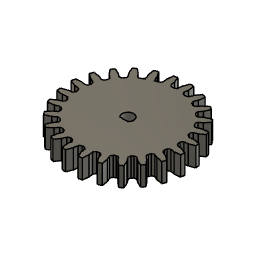
шестерня двигателя (Autodesk Fusion 360 design; units mm, degrees)
Autodesk Fusion 360 part; units mm, degrees
(part 1 of 2)
sketch "Sketch1" plane through (0, 0, 0) normal (0, 1, 0) x (1, 0, 0)
  circle A0 centre (0, 0) radius 12.5
  line L0 (0, 0) -> (0, 12.5)
  line L1 (0, 12.5) -> (0, 15.5)
  line L2 (0, 12.5) -> (-1.5967, 12.3976)
  line L3 (0, 0) -> (-1.5967, 12.3976)
  line L4 (-1.5967, 12.3976) -> (-1.9799, 15.373)
  line L5 (-1.9799, 15.373) -> (-3.666, 15.1559)
  line L6 (0, 12.5) -> (1.5967, 12.3976)
  line L7 (-3.666, 15.1559) -> (-3.268, 12.0653)
  line L8 (-4.751, 11.5619) -> (-5.8913, 14.3368)
  line L9 (-5.8913, 14.3368) -> (-7.4637, 13.6906)
  line L10 (-7.4637, 13.6906) -> (-6.2793, 10.8083)
  line L11 (-7.5816, 9.9383) -> (-9.4012, 12.3235)
  line L12 (-9.4012, 12.3235) -> (-10.7528, 11.2924)
  line L13 (-10.7528, 11.2924) -> (-8.8628, 8.8148)
  line L14 (-9.8955, 7.6374) -> (-12.2704, 9.4703)
  line L15 (-12.2704, 9.4703) -> (-13.3091, 8.1246)
  line L16 (-13.3091, 8.1246) -> (-10.8422, 6.2206)
  line L17 (-11.535, 4.816) -> (-14.3034, 5.9718)
  line L18 (-14.3034, 5.9718) -> (-14.9584, 4.4031)
  line L19 (-14.9584, 4.4031) -> (-12.0828, 3.2025)
  line L20 (-12.3884, 1.6664) -> (-15.3616, 2.0664)
  line L21 (-15.3616, 2.0664) -> (-15.5883, 0.3815)
  line L22 (-15.5883, 0.3815) -> (-12.5, -0.0339)
  line L23 (-12.3976, -1.5967) -> (-15.373, -1.9799)
  line L24 (-15.373, -1.9799) -> (-15.1559, -3.666)
  line L25 (-15.1559, -3.666) -> (-12.0653, -3.268)
  line L26 (-11.5619, -4.751) -> (-14.3368, -5.8913)
  line L27 (-14.3368, -5.8913) -> (-13.6906, -7.4637)
  line L28 (-13.6906, -7.4637) -> (-10.8083, -6.2793)
  line L29 (-9.9383, -7.5816) -> (-12.3235, -9.4012)
  line L30 (-12.3235, -9.4012) -> (-11.2924, -10.7528)
  line L31 (-11.2924, -10.7528) -> (-8.8148, -8.8628)
  line L32 (-7.6374, -9.8955) -> (-9.4703, -12.2704)
  line L33 (-9.4703, -12.2704) -> (-8.1246, -13.3091)
  line L34 (-8.1246, -13.3091) -> (-6.2206, -10.8422)
  line L35 (-4.816, -11.535) -> (-5.9718, -14.3034)
  line L36 (-5.9718, -14.3034) -> (-4.4031, -14.9584)
  line L37 (-4.4031, -14.9584) -> (-3.2025, -12.0828)
  line L38 (-1.6664, -12.3884) -> (-2.0664, -15.3616)
  line L39 (-2.0664, -15.3616) -> (-0.3815, -15.5883)
  line L40 (-0.3815, -15.5883) -> (0.0339, -12.5)
  line L41 (1.5967, -12.3976) -> (1.9799, -15.373)
  line L42 (1.9799, -15.373) -> (3.666, -15.1559)
  line L43 (3.666, -15.1559) -> (3.268, -12.0653)
  line L44 (4.751, -11.5619) -> (5.8913, -14.3368)
  line L45 (5.8913, -14.3368) -> (7.4637, -13.6906)
  line L46 (7.4637, -13.6906) -> (6.2793, -10.8083)
  line L47 (7.5816, -9.9383) -> (9.4012, -12.3235)
  line L48 (9.4012, -12.3235) -> (10.7528, -11.2924)
  line L49 (10.7528, -11.2924) -> (8.8628, -8.8148)
  line L50 (9.8955, -7.6374) -> (12.2704, -9.4703)
  line L51 (12.2704, -9.4703) -> (13.3091, -8.1246)
  line L52 (13.3091, -8.1246) -> (10.8422, -6.2206)
  line L53 (11.535, -4.816) -> (14.3034, -5.9718)
  line L54 (14.3034, -5.9718) -> (14.9584, -4.4031)
  line L55 (14.9584, -4.4031) -> (12.0828, -3.2025)
  line L56 (12.3884, -1.6664) -> (15.3616, -2.0664)
  line L57 (15.3616, -2.0664) -> (15.5883, -0.3815)
  line L58 (15.5883, -0.3815) -> (12.5, 0.0339)
  line L59 (12.3976, 1.5967) -> (15.373, 1.9799)
  line L60 (15.373, 1.9799) -> (15.1559, 3.666)
  line L61 (15.1559, 3.666) -> (12.0653, 3.268)
  line L62 (11.5619, 4.751) -> (14.3368, 5.8913)
  line L63 (14.3368, 5.8913) -> (13.6906, 7.4637)
  line L64 (13.6906, 7.4637) -> (10.8083, 6.2793)
  line L65 (9.9383, 7.5816) -> (12.3235, 9.4012)
  line L66 (12.3235, 9.4012) -> (11.2924, 10.7528)
  line L67 (11.2924, 10.7528) -> (8.8148, 8.8628)
  line L68 (7.6374, 9.8955) -> (9.4703, 12.2704)
  line L69 (9.4703, 12.2704) -> (8.1246, 13.3091)
  line L70 (8.1246, 13.3091) -> (6.2206, 10.8422)
  line L71 (4.816, 11.535) -> (5.9718, 14.3034)
  line L72 (5.9718, 14.3034) -> (4.4031, 14.9584)
  line L73 (4.4031, 14.9584) -> (3.2025, 12.0828)
  line L74 (1.6664, 12.3884) -> (2.0664, 15.3616)
  line L75 (2.0664, 15.3616) -> (0.3815, 15.5883)
  line L76 (0.3815, 15.5883) -> (-0.0339, 12.5)
  line L77 (-3.268, 12.0653) -> (-3.467, 13.6106)
  line L78 (-2.823, 15.2644) -> (-3.3189, 15.2006)
  line L79 (-2.823, 15.2644) -> (-2.3271, 15.3283)
  line L80 (-3.3189, 15.2006) -> (-3.467, 13.6106)
  line L81 (-2.3271, 15.3283) -> (-1.7883, 13.8853)
  line L82 (-6.215, 14.2037) -> (-5.3212, 12.9493)
  line L83 (-7.14, 13.8236) -> (-6.8715, 12.2495)
  line L84 (-9.6795, 12.1112) -> (-8.4914, 11.1309)
  line L85 (-10.4745, 11.5047) -> (-9.8078, 10.0536)
  line L86 (-12.4842, 9.1933) -> (-11.0829, 8.5539)
  line L87 (-13.0952, 8.4016) -> (-12.0756, 7.1726)
  line L88 (-14.4382, 5.6489) -> (-12.9192, 5.3939)
  line L89 (-14.8235, 4.7261) -> (-13.5206, 3.8028)
  line L90 (-15.4083, 1.7195) -> (-13.875, 1.8664)
  line L91 (-15.5416, 0.7284) -> (-14.0441, 0.1738)
  line L92 (-15.3283, -2.3271) -> (-13.8853, -1.7883)
  line L93 (-15.2006, -3.3189) -> (-13.6106, -3.467)
  line L94 (-14.2037, -6.215) -> (-12.9493, -5.3212)
  line L95 (-13.8236, -7.14) -> (-12.2495, -6.8715)
  line L96 (-12.1112, -9.6795) -> (-11.1309, -8.4914)
  line L97 (-11.5047, -10.4745) -> (-10.0536, -9.8078)
  line L98 (-9.1933, -12.4842) -> (-8.5539, -11.0829)
  line L99 (-8.4016, -13.0952) -> (-7.1726, -12.0756)
  line L100 (-5.6489, -14.4382) -> (-5.3939, -12.9192)
  line L101 (-4.7261, -14.8235) -> (-3.8028, -13.5206)
  line L102 (-1.7195, -15.4083) -> (-1.8664, -13.875)
  line L103 (-0.7284, -15.5416) -> (-0.1738, -14.0441)
  line L104 (2.3271, -15.3283) -> (1.7883, -13.8853)
  line L105 (3.3189, -15.2006) -> (3.467, -13.6106)
  line L106 (6.215, -14.2037) -> (5.3212, -12.9493)
  line L107 (7.14, -13.8236) -> (6.8715, -12.2495)
  line L108 (9.6795, -12.1112) -> (8.4914, -11.1309)
  line L109 (10.4745, -11.5047) -> (9.8078, -10.0536)
  line L110 (12.4842, -9.1933) -> (11.0829, -8.5539)
  line L111 (13.0952, -8.4016) -> (12.0756, -7.1726)
  line L112 (14.4382, -5.6489) -> (12.9192, -5.3939)
  line L113 (14.8235, -4.7261) -> (13.5206, -3.8028)
  line L114 (15.4083, -1.7195) -> (13.875, -1.8664)
  line L115 (15.5416, -0.7284) -> (14.0441, -0.1738)
  line L116 (15.3283, 2.3271) -> (13.8853, 1.7883)
  line L117 (15.2006, 3.3189) -> (13.6106, 3.467)
  line L118 (14.2037, 6.215) -> (12.9493, 5.3212)
  line L119 (13.8236, 7.14) -> (12.2495, 6.8715)
  line L120 (12.1112, 9.6795) -> (11.1309, 8.4914)
  line L121 (11.5047, 10.4745) -> (10.0536, 9.8078)
  line L122 (9.1933, 12.4842) -> (8.5539, 11.0829)
  line L123 (8.4016, 13.0952) -> (7.1726, 12.0756)
  line L124 (5.6489, 14.4382) -> (5.3939, 12.9192)
  line L125 (4.7261, 14.8235) -> (3.8028, 13.5206)
  line L126 (1.7195, 15.4083) -> (1.8664, 13.875)
  line L127 (0.7284, 15.5416) -> (0.1738, 14.0441)
  line L128 (-4.751, 11.5619) -> (-4.9411, 12.0244)
  line L129 (-4.751, 11.5619) -> (-4.2886, 11.7519)
  line L130 (-4.9411, 12.0244) -> (-4.2886, 11.7519)
  line L131 (-4.6148, 11.8882) -> (-4.6534, 11.7959)
  spline S0 degree 5 poles (-4.9411, 12.0244) (-4.931, 12.0121) (-4.9104, 11.9882) (-4.8789, 11.954) (-4.8353, 11.9119) (-4.778, 11.8656) (-4.7177, 11.8261) (-4.6541, 11.7939) (-4.5872, 11.7695) (-4.517, 11.7524) (-4.4438, 11.7421) (-4.383, 11.7389) (-4.3362, 11.7391) (-4.3045, 11.7404) (-4.2886, 11.7413) knots 0 0 0 0 0 0 0.1 0.2 0.3 0.4 0.5 0.6 0.7 0.8 0.9 1 1 1 1 1 1
  line L132 (-6.2793, 10.8083) -> (-6.4694, 11.2708)
  line L133 (-6.2793, 10.8083) -> (-6.7117, 10.5572)
  line L134 (-6.4694, 11.2708) -> (-6.7117, 10.5572)
  line L135 (-6.5905, 10.914) -> (-6.4958, 10.8818)
  spline S1 degree 5 poles (-6.4694, 11.2708) (-6.467, 11.2543) (-6.4628, 11.2214) (-6.4584, 11.1727) (-6.4566, 11.1087) (-6.4612, 11.0305) (-6.4735, 10.9543) (-6.494, 10.8803) (-6.523, 10.8086) (-6.5603, 10.739) (-6.6051, 10.6714) (-6.6465, 10.6188) (-6.6805, 10.5801) (-6.7045, 10.5547) (-6.7168, 10.542) knots 0 0 0 0 0 0 0.1 0.2 0.3 0.4 0.5 0.6 0.7 0.8 0.9 1 1 1 1 1 1
  spline S2 degree 5 poles (-7.8849, 10.3358) (-7.8719, 10.3266) (-7.8459, 10.3088) (-7.8066, 10.2839) (-7.7535, 10.2546) (-7.6862, 10.2246) (-7.6177, 10.2021) (-7.548, 10.1875) (-7.477, 10.1812) (-7.4048, 10.1828) (-7.3314, 10.1918) (-7.2719, 10.2045) (-7.2268, 10.2168) (-7.1965, 10.2262) (-7.1813, 10.2313) knots 0 0 0 0 0 0 0.1 0.2 0.3 0.4 0.5 0.6 0.7 0.8 0.9 1 1 1 1 1 1
  spline S3 degree 5 poles (-9.166, 9.2124) (-9.1594, 9.197) (-9.1469, 9.1664) (-9.1301, 9.1204) (-9.1117, 9.0591) (-9.096, 8.9823) (-9.0881, 8.9056) (-9.0888, 8.8288) (-9.0982, 8.752) (-9.1162, 8.6752) (-9.142, 8.5983) (-9.1684, 8.5367) (-9.1913, 8.4906) (-9.2078, 8.4598) (-9.2164, 8.4444) knots 0 0 0 0 0 0 0.1 0.2 0.3 0.4 0.5 0.6 0.7 0.8 0.9 1 1 1 1 1 1
  spline S4 degree 5 poles (-10.2913, 7.9429) (-10.2764, 7.9373) (-10.2466, 7.9268) (-10.2022, 7.913) (-10.1434, 7.8984) (-10.0706, 7.8869) (-9.9987, 7.8828) (-9.9276, 7.8868) (-9.8573, 7.8991) (-9.788, 7.9194) (-9.7194, 7.9471) (-9.6652, 7.9747) (-9.6248, 7.9982) (-9.598, 8.0152) (-9.5847, 8.024) knots 0 0 0 0 0 0 0.1 0.2 0.3 0.4 0.5 0.6 0.7 0.8 0.9 1 1 1 1 1 1
  spline S5 degree 5 poles (-11.238, 6.5261) (-11.2277, 6.513) (-11.2076, 6.4867) (-11.1795, 6.4466) (-11.1459, 6.3921) (-11.1109, 6.3221) (-11.0834, 6.25) (-11.0641, 6.1756) (-11.0534, 6.099) (-11.0509, 6.0201) (-11.0559, 5.9392) (-11.0655, 5.8729) (-11.0756, 5.8224) (-11.0836, 5.7884) (-11.0879, 5.7713) knots 0 0 0 0 0 0 0.1 0.2 0.3 0.4 0.5 0.6 0.7 0.8 0.9 1 1 1 1 1 1
  spline S6 degree 5 poles (-11.9964, 5.0086) (-11.9806, 5.0071) (-11.9491, 5.0047) (-11.9026, 5.0029) (-11.842, 5.0039) (-11.7688, 5.0117) (-11.6982, 5.0264) (-11.6305, 5.0486) (-11.5659, 5.0786) (-11.5042, 5.1162) (-11.4451, 5.1607) (-11.3998, 5.2014) (-11.3669, 5.2346) (-11.3455, 5.2579) (-11.3348, 5.2699) knots 0 0 0 0 0 0 0.1 0.2 0.3 0.4 0.5 0.6 0.7 0.8 0.9 1 1 1 1 1 1
  spline S7 degree 5 poles (-12.5442, 3.3951) (-12.5308, 3.3852) (-12.5046, 3.3649) (-12.4671, 3.3335) (-12.4205, 3.2895) (-12.3685, 3.2309) (-12.3233, 3.1684) (-12.2855, 3.1016) (-12.2553, 3.0303) (-12.2325, 2.9548) (-12.2164, 2.8753) (-12.2085, 2.8088) (-12.2051, 2.7574) (-12.2041, 2.7225) (-12.2038, 2.7049) knots 0 0 0 0 0 0 0.1 0.2 0.3 0.4 0.5 0.6 0.7 0.8 0.9 1 1 1 1 1 1
  spline S8 degree 5 poles (-12.884, 1.7331) (-12.8683, 1.7357) (-12.8373, 1.7415) (-12.7919, 1.7518) (-12.7337, 1.7685) (-12.6649, 1.7949) (-12.6005, 1.8274) (-12.5409, 1.8664) (-12.4862, 1.9121) (-12.4363, 1.9644) (-12.3908, 2.0226) (-12.3576, 2.0737) (-12.3344, 2.1143) (-12.3197, 2.1423) (-12.3126, 2.1566) knots 0 0 0 0 0 0 0.1 0.2 0.3 0.4 0.5 0.6 0.7 0.8 0.9 1 1 1 1 1 1
  spline S9 degree 5 poles (-12.9955, 0.0328) (-12.98, 0.0266) (-12.9494, 0.0138) (-12.905, -0.0068) (-12.8487, -0.0372) (-12.7833, -0.0804) (-12.7235, -0.1291) (-12.6697, -0.1838) (-12.622, -0.2448) (-12.5804, -0.3119) (-12.5443, -0.3845) (-12.5194, -0.4467) (-12.5029, -0.4955) (-12.4929, -0.5289) (-12.4881, -0.5459) knots 0 0 0 0 0 0 0.1 0.2 0.3 0.4 0.5 0.6 0.7 0.8 0.9 1 1 1 1 1 1
  spline S10 degree 5 poles (-12.8935, -1.6606) (-12.879, -1.654) (-12.8506, -1.6403) (-12.8094, -1.6187) (-12.7575, -1.5875) (-12.6979, -1.5441) (-12.6441, -1.4961) (-12.5966, -1.443) (-12.5557, -1.3847) (-12.521, -1.3213) (-12.4921, -1.2533) (-12.4733, -1.1954) (-12.4614, -1.1502) (-12.4544, -1.1192) (-12.4512, -1.1036) knots 0 0 0 0 0 0 0.1 0.2 0.3 0.4 0.5 0.6 0.7 0.8 0.9 1 1 1 1 1 1
  spline S11 degree 5 poles (-12.5612, -3.3318) (-12.5446, -3.3338) (-12.5118, -3.3382) (-12.4635, -3.3467) (-12.4012, -3.3614) (-12.3269, -3.3862) (-12.2565, -3.4177) (-12.1904, -3.4567) (-12.1286, -3.5033) (-12.071, -3.5573) (-12.0173, -3.6181) (-11.9772, -3.6717) (-11.9487, -3.7146) (-11.9303, -3.7443) (-11.9213, -3.7594) knots 0 0 0 0 0 0 0.1 0.2 0.3 0.4 0.5 0.6 0.7 0.8 0.9 1 1 1 1 1 1
  spline S12 degree 5 poles (-12.0244, -4.9411) (-12.0121, -4.931) (-11.9882, -4.9104) (-11.954, -4.8789) (-11.9119, -4.8353) (-11.8656, -4.778) (-11.8261, -4.7177) (-11.7939, -4.6541) (-11.7695, -4.5872) (-11.7524, -4.517) (-11.7421, -4.4438) (-11.7389, -4.383) (-11.7391, -4.3362) (-11.7404, -4.3045) (-11.7413, -4.2886) knots 0 0 0 0 0 0 0.1 0.2 0.3 0.4 0.5 0.6 0.7 0.8 0.9 1 1 1 1 1 1
  spline S13 degree 5 poles (-11.2708, -6.4694) (-11.2543, -6.467) (-11.2214, -6.4628) (-11.1727, -6.4584) (-11.1087, -6.4566) (-11.0305, -6.4612) (-10.9543, -6.4735) (-10.8803, -6.494) (-10.8086, -6.523) (-10.739, -6.5603) (-10.6714, -6.6051) (-10.6188, -6.6465) (-10.5801, -6.6805) (-10.5547, -6.7045) (-10.542, -6.7168) knots 0 0 0 0 0 0 0.1 0.2 0.3 0.4 0.5 0.6 0.7 0.8 0.9 1 1 1 1 1 1
  spline S14 degree 5 poles (-10.3358, -7.8849) (-10.3266, -7.8719) (-10.3088, -7.8459) (-10.2839, -7.8066) (-10.2546, -7.7535) (-10.2246, -7.6862) (-10.2021, -7.6177) (-10.1875, -7.548) (-10.1812, -7.477) (-10.1828, -7.4048) (-10.1918, -7.3314) (-10.2045, -7.2719) (-10.2168, -7.2268) (-10.2262, -7.1965) (-10.2313, -7.1813) knots 0 0 0 0 0 0 0.1 0.2 0.3 0.4 0.5 0.6 0.7 0.8 0.9 1 1 1 1 1 1
  spline S15 degree 5 poles (-9.2124, -9.166) (-9.197, -9.1594) (-9.1664, -9.1469) (-9.1204, -9.1301) (-9.0591, -9.1117) (-8.9823, -9.096) (-8.9056, -9.0881) (-8.8288, -9.0888) (-8.752, -9.0982) (-8.6752, -9.1162) (-8.5983, -9.142) (-8.5367, -9.1684) (-8.4906, -9.1913) (-8.4598, -9.2078) (-8.4444, -9.2164) knots 0 0 0 0 0 0 0.1 0.2 0.3 0.4 0.5 0.6 0.7 0.8 0.9 1 1 1 1 1 1
  spline S16 degree 5 poles (-7.9429, -10.2913) (-7.9373, -10.2764) (-7.9268, -10.2466) (-7.913, -10.2022) (-7.8984, -10.1434) (-7.8869, -10.0706) (-7.8828, -9.9987) (-7.8868, -9.9276) (-7.8991, -9.8573) (-7.9194, -9.788) (-7.9471, -9.7194) (-7.9747, -9.6652) (-7.9982, -9.6248) (-8.0152, -9.598) (-8.024, -9.5847) knots 0 0 0 0 0 0 0.1 0.2 0.3 0.4 0.5 0.6 0.7 0.8 0.9 1 1 1 1 1 1
  spline S17 degree 5 poles (-6.5261, -11.238) (-6.513, -11.2277) (-6.4867, -11.2076) (-6.4466, -11.1795) (-6.3921, -11.1459) (-6.3221, -11.1109) (-6.25, -11.0834) (-6.1756, -11.0641) (-6.099, -11.0534) (-6.0201, -11.0509) (-5.9392, -11.0559) (-5.8729, -11.0655) (-5.8224, -11.0756) (-5.7884, -11.0836) (-5.7713, -11.0879) knots 0 0 0 0 0 0 0.1 0.2 0.3 0.4 0.5 0.6 0.7 0.8 0.9 1 1 1 1 1 1
  spline S18 degree 5 poles (-5.0086, -11.9964) (-5.0071, -11.9806) (-5.0047, -11.9491) (-5.0029, -11.9026) (-5.0039, -11.842) (-5.0117, -11.7688) (-5.0264, -11.6982) (-5.0486, -11.6305) (-5.0786, -11.5659) (-5.1162, -11.5042) (-5.1607, -11.4451) (-5.2014, -11.3998) (-5.2346, -11.3669) (-5.2579, -11.3455) (-5.2699, -11.3348) knots 0 0 0 0 0 0 0.1 0.2 0.3 0.4 0.5 0.6 0.7 0.8 0.9 1 1 1 1 1 1
  spline S19 degree 5 poles (-3.3951, -12.5442) (-3.3852, -12.5308) (-3.3649, -12.5046) (-3.3335, -12.4671) (-3.2895, -12.4205) (-3.2309, -12.3685) (-3.1684, -12.3233) (-3.1016, -12.2855) (-3.0303, -12.2553) (-2.9548, -12.2325) (-2.8753, -12.2164) (-2.8088, -12.2085) (-2.7574, -12.2051) (-2.7225, -12.2041) (-2.7049, -12.2038) knots 0 0 0 0 0 0 0.1 0.2 0.3 0.4 0.5 0.6 0.7 0.8 0.9 1 1 1 1 1 1
  spline S20 degree 5 poles (-1.7331, -12.884) (-1.7357, -12.8683) (-1.7415, -12.8373) (-1.7518, -12.7919) (-1.7685, -12.7337) (-1.7949, -12.6649) (-1.8274, -12.6005) (-1.8664, -12.5409) (-1.9121, -12.4862) (-1.9644, -12.4363) (-2.0226, -12.3908) (-2.0737, -12.3576) (-2.1143, -12.3344) (-2.1423, -12.3197) (-2.1566, -12.3126) knots 0 0 0 0 0 0 0.1 0.2 0.3 0.4 0.5 0.6 0.7 0.8 0.9 1 1 1 1 1 1
  spline S21 degree 5 poles (-0.0328, -12.9955) (-0.0266, -12.98) (-0.0138, -12.9494) (0.0068, -12.905) (0.0372, -12.8487) (0.0804, -12.7833) (0.1291, -12.7235) (0.1838, -12.6697) (0.2448, -12.622) (0.3119, -12.5804) (0.3845, -12.5443) (0.4467, -12.5194) (0.4955, -12.5029) (0.5289, -12.4929) (0.5459, -12.4881) knots 0 0 0 0 0 0 0.1 0.2 0.3 0.4 0.5 0.6 0.7 0.8 0.9 1 1 1 1 1 1
  spline S22 degree 5 poles (1.6606, -12.8935) (1.654, -12.879) (1.6403, -12.8506) (1.6187, -12.8094) (1.5875, -12.7575) (1.5441, -12.6979) (1.4961, -12.6441) (1.443, -12.5966) (1.3847, -12.5557) (1.3213, -12.521) (1.2533, -12.4921) (1.1954, -12.4733) (1.1502, -12.4614) (1.1192, -12.4544) (1.1036, -12.4512) knots 0 0 0 0 0 0 0.1 0.2 0.3 0.4 0.5 0.6 0.7 0.8 0.9 1 1 1 1 1 1
  spline S23 degree 5 poles (3.3318, -12.5612) (3.3338, -12.5446) (3.3382, -12.5118) (3.3467, -12.4635) (3.3614, -12.4012) (3.3862, -12.3269) (3.4177, -12.2565) (3.4567, -12.1904) (3.5033, -12.1286) (3.5573, -12.071) (3.6181, -12.0173) (3.6717, -11.9772) (3.7146, -11.9487) (3.7443, -11.9303) (3.7594, -11.9213) knots 0 0 0 0 0 0 0.1 0.2 0.3 0.4 0.5 0.6 0.7 0.8 0.9 1 1 1 1 1 1
  spline S24 degree 5 poles (4.9411, -12.0244) (4.931, -12.0121) (4.9104, -11.9882) (4.8789, -11.954) (4.8353, -11.9119) (4.778, -11.8656) (4.7177, -11.8261) (4.6541, -11.7939) (4.5872, -11.7695) (4.517, -11.7524) (4.4438, -11.7421) (4.383, -11.7389) (4.3362, -11.7391) (4.3045, -11.7404) (4.2886, -11.7413) knots 0 0 0 0 0 0 0.1 0.2 0.3 0.4 0.5 0.6 0.7 0.8 0.9 1 1 1 1 1 1
  spline S25 degree 5 poles (6.4694, -11.2708) (6.467, -11.2543) (6.4628, -11.2214) (6.4584, -11.1727) (6.4566, -11.1087) (6.4612, -11.0305) (6.4735, -10.9543) (6.494, -10.8803) (6.523, -10.8086) (6.5603, -10.739) (6.6051, -10.6714) (6.6465, -10.6188) (6.6805, -10.5801) (6.7045, -10.5547) (6.7168, -10.542) knots 0 0 0 0 0 0 0.1 0.2 0.3 0.4 0.5 0.6 0.7 0.8 0.9 1 1 1 1 1 1
  spline S26 degree 5 poles (7.8849, -10.3358) (7.8719, -10.3266) (7.8459, -10.3088) (7.8066, -10.2839) (7.7535, -10.2546) (7.6862, -10.2246) (7.6177, -10.2021) (7.548, -10.1875) (7.477, -10.1812) (7.4048, -10.1828) (7.3314, -10.1918) (7.2719, -10.2045) (7.2268, -10.2168) (7.1965, -10.2262) (7.1813, -10.2313) knots 0 0 0 0 0 0 0.1 0.2 0.3 0.4 0.5 0.6 0.7 0.8 0.9 1 1 1 1 1 1
  spline S27 degree 5 poles (9.166, -9.2124) (9.1594, -9.197) (9.1469, -9.1664) (9.1301, -9.1204) (9.1117, -9.0591) (9.096, -8.9823) (9.0881, -8.9056) (9.0888, -8.8288) (9.0982, -8.752) (9.1162, -8.6752) (9.142, -8.5983) (9.1684, -8.5367) (9.1913, -8.4906) (9.2078, -8.4598) (9.2164, -8.4444) knots 0 0 0 0 0 0 0.1 0.2 0.3 0.4 0.5 0.6 0.7 0.8 0.9 1 1 1 1 1 1
  spline S28 degree 5 poles (10.2913, -7.9429) (10.2764, -7.9373) (10.2466, -7.9268) (10.2022, -7.913) (10.1434, -7.8984) (10.0706, -7.8869) (9.9987, -7.8828) (9.9276, -7.8868) (9.8573, -7.8991) (9.788, -7.9194) (9.7194, -7.9471) (9.6652, -7.9747) (9.6248, -7.9982) (9.598, -8.0152) (9.5847, -8.024) knots 0 0 0 0 0 0 0.1 0.2 0.3 0.4 0.5 0.6 0.7 0.8 0.9 1 1 1 1 1 1
  spline S29 degree 5 poles (11.238, -6.5261) (11.2277, -6.513) (11.2076, -6.4867) (11.1795, -6.4466) (11.1459, -6.3921) (11.1109, -6.3221) (11.0834, -6.25) (11.0641, -6.1756) (11.0534, -6.099) (11.0509, -6.0201) (11.0559, -5.9392) (11.0655, -5.8729) (11.0756, -5.8224) (11.0836, -5.7884) (11.0879, -5.7713) knots 0 0 0 0 0 0 0.1 0.2 0.3 0.4 0.5 0.6 0.7 0.8 0.9 1 1 1 1 1 1
  spline S30 degree 5 poles (11.9964, -5.0086) (11.9806, -5.0071) (11.9491, -5.0047) (11.9026, -5.0029) (11.842, -5.0039) (11.7688, -5.0117) (11.6982, -5.0264) (11.6305, -5.0486) (11.5659, -5.0786) (11.5042, -5.1162) (11.4451, -5.1607) (11.3998, -5.2014) (11.3669, -5.2346) (11.3455, -5.2579) (11.3348, -5.2699) knots 0 0 0 0 0 0 0.1 0.2 0.3 0.4 0.5 0.6 0.7 0.8 0.9 1 1 1 1 1 1
  spline S31 degree 5 poles (12.5442, -3.3951) (12.5308, -3.3852) (12.5046, -3.3649) (12.4671, -3.3335) (12.4205, -3.2895) (12.3685, -3.2309) (12.3233, -3.1684) (12.2855, -3.1016) (12.2553, -3.0303) (12.2325, -2.9548) (12.2164, -2.8753) (12.2085, -2.8088) (12.2051, -2.7574) (12.2041, -2.7225) (12.2038, -2.7049) knots 0 0 0 0 0 0 0.1 0.2 0.3 0.4 0.5 0.6 0.7 0.8 0.9 1 1 1 1 1 1
  spline S32 degree 5 poles (12.884, -1.7331) (12.8683, -1.7357) (12.8373, -1.7415) (12.7919, -1.7518) (12.7337, -1.7685) (12.6649, -1.7949) (12.6005, -1.8274) (12.5409, -1.8664) (12.4862, -1.9121) (12.4363, -1.9644) (12.3908, -2.0226) (12.3576, -2.0737) (12.3344, -2.1143) (12.3197, -2.1423) (12.3126, -2.1566) knots 0 0 0 0 0 0 0.1 0.2 0.3 0.4 0.5 0.6 0.7 0.8 0.9 1 1 1 1 1 1
  spline S33 degree 5 poles (12.9955, -0.0328) (12.98, -0.0266) (12.9494, -0.0138) (12.905, 0.0068) (12.8487, 0.0372) (12.7833, 0.0804) (12.7235, 0.1291) (12.6697, 0.1838) (12.622, 0.2448) (12.5804, 0.3119) (12.5443, 0.3845) (12.5194, 0.4467) (12.5029, 0.4955) (12.4929, 0.5289) (12.4881, 0.5459) knots 0 0 0 0 0 0 0.1 0.2 0.3 0.4 0.5 0.6 0.7 0.8 0.9 1 1 1 1 1 1
  spline S34 degree 5 poles (12.8935, 1.6606) (12.879, 1.654) (12.8506, 1.6403) (12.8094, 1.6187) (12.7575, 1.5875) (12.6979, 1.5441) (12.6441, 1.4961) (12.5966, 1.443) (12.5557, 1.3847) (12.521, 1.3213) (12.4921, 1.2533) (12.4733, 1.1954) (12.4614, 1.1502) (12.4544, 1.1192) (12.4512, 1.1036) knots 0 0 0 0 0 0 0.1 0.2 0.3 0.4 0.5 0.6 0.7 0.8 0.9 1 1 1 1 1 1
  spline S35 degree 5 poles (12.5612, 3.3318) (12.5446, 3.3338) (12.5118, 3.3382) (12.4635, 3.3467) (12.4012, 3.3614) (12.3269, 3.3862) (12.2565, 3.4177) (12.1904, 3.4567) (12.1286, 3.5033) (12.071, 3.5573) (12.0173, 3.6181) (11.9772, 3.6717) (11.9487, 3.7146) (11.9303, 3.7443) (11.9213, 3.7594) knots 0 0 0 0 0 0 0.1 0.2 0.3 0.4 0.5 0.6 0.7 0.8 0.9 1 1 1 1 1 1
  spline S36 degree 5 poles (12.0244, 4.9411) (12.0121, 4.931) (11.9882, 4.9104) (11.954, 4.8789) (11.9119, 4.8353) (11.8656, 4.778) (11.8261, 4.7177) (11.7939, 4.6541) (11.7695, 4.5872) (11.7524, 4.517) (11.7421, 4.4438) (11.7389, 4.383) (11.7391, 4.3362) (11.7404, 4.3045) (11.7413, 4.2886) knots 0 0 0 0 0 0 0.1 0.2 0.3 0.4 0.5 0.6 0.7 0.8 0.9 1 1 1 1 1 1
  spline S37 degree 5 poles (11.2708, 6.4694) (11.2543, 6.467) (11.2214, 6.4628) (11.1727, 6.4584) (11.1087, 6.4566) (11.0305, 6.4612) (10.9543, 6.4735) (10.8803, 6.494) (10.8086, 6.523) (10.739, 6.5603) (10.6714, 6.6051) (10.6188, 6.6465) (10.5801, 6.6805) (10.5547, 6.7045) (10.542, 6.7168) knots 0 0 0 0 0 0 0.1 0.2 0.3 0.4 0.5 0.6 0.7 0.8 0.9 1 1 1 1 1 1
  spline S38 degree 5 poles (10.3358, 7.8849) (10.3266, 7.8719) (10.3088, 7.8459) (10.2839, 7.8066) (10.2546, 7.7535) (10.2246, 7.6862) (10.2021, 7.6177) (10.1875, 7.548) (10.1812, 7.477) (10.1828, 7.4048) (10.1918, 7.3314) (10.2045, 7.2719) (10.2168, 7.2268) (10.2262, 7.1965) (10.2313, 7.1813) knots 0 0 0 0 0 0 0.1 0.2 0.3 0.4 0.5 0.6 0.7 0.8 0.9 1 1 1 1 1 1
  spline S39 degree 5 poles (9.2124, 9.166) (9.197, 9.1594) (9.1664, 9.1469) (9.1204, 9.1301) (9.0591, 9.1117) (8.9823, 9.096) (8.9056, 9.0881) (8.8288, 9.0888) (8.752, 9.0982) (8.6752, 9.1162) (8.5983, 9.142) (8.5367, 9.1684) (8.4906, 9.1913) (8.4598, 9.2078) (8.4444, 9.2164) knots 0 0 0 0 0 0 0.1 0.2 0.3 0.4 0.5 0.6 0.7 0.8 0.9 1 1 1 1 1 1
  spline S40 degree 5 poles (7.9429, 10.2913) (7.9373, 10.2764) (7.9268, 10.2466) (7.913, 10.2022) (7.8984, 10.1434) (7.8869, 10.0706) (7.8828, 9.9987) (7.8868, 9.9276) (7.8991, 9.8573) (7.9194, 9.788) (7.9471, 9.7194) (7.9747, 9.6652) (7.9982, 9.6248) (8.0152, 9.598) (8.024, 9.5847) knots 0 0 0 0 0 0 0.1 0.2 0.3 0.4 0.5 0.6 0.7 0.8 0.9 1 1 1 1 1 1
  spline S41 degree 5 poles (6.5261, 11.238) (6.513, 11.2277) (6.4867, 11.2076) (6.4466, 11.1795) (6.3921, 11.1459) (6.3221, 11.1109) (6.25, 11.0834) (6.1756, 11.0641) (6.099, 11.0534) (6.0201, 11.0509) (5.9392, 11.0559) (5.8729, 11.0655) (5.8224, 11.0756) (5.7884, 11.0836) (5.7713, 11.0879) knots 0 0 0 0 0 0 0.1 0.2 0.3 0.4 0.5 0.6 0.7 0.8 0.9 1 1 1 1 1 1
  spline S42 degree 5 poles (5.0086, 11.9964) (5.0071, 11.9806) (5.0047, 11.9491) (5.0029, 11.9026) (5.0039, 11.842) (5.0117, 11.7688) (5.0264, 11.6982) (5.0486, 11.6305) (5.0786, 11.5659) (5.1162, 11.5042) (5.1607, 11.4451) (5.2014, 11.3998) (5.2346, 11.3669) (5.2579, 11.3455) (5.2699, 11.3348) knots 0 0 0 0 0 0 0.1 0.2 0.3 0.4 0.5 0.6 0.7 0.8 0.9 1 1 1 1 1 1
  spline S43 degree 5 poles (3.3951, 12.5442) (3.3852, 12.5308) (3.3649, 12.5046) (3.3335, 12.4671) (3.2895, 12.4205) (3.2309, 12.3685) (3.1684, 12.3233) (3.1016, 12.2855) (3.0303, 12.2553) (2.9548, 12.2325) (2.8753, 12.2164) (2.8088, 12.2085) (2.7574, 12.2051) (2.7225, 12.2041) (2.7049, 12.2038) knots 0 0 0 0 0 0 0.1 0.2 0.3 0.4 0.5 0.6 0.7 0.8 0.9 1 1 1 1 1 1
  spline S44 degree 5 poles (1.7331, 12.884) (1.7357, 12.8683) (1.7415, 12.8373) (1.7518, 12.7919) (1.7685, 12.7337) (1.7949, 12.6649) (1.8274, 12.6005) (1.8664, 12.5409) (1.9121, 12.4862) (1.9644, 12.4363) (2.0226, 12.3908) (2.0737, 12.3576) (2.1143, 12.3344) (2.1423, 12.3197) (2.1566, 12.3126) knots 0 0 0 0 0 0 0.1 0.2 0.3 0.4 0.5 0.6 0.7 0.8 0.9 1 1 1 1 1 1
  spline S45 degree 5 poles (0.0328, 12.9955) (0.0266, 12.98) (0.0138, 12.9494) (-0.0068, 12.905) (-0.0372, 12.8487) (-0.0804, 12.7833) (-0.1291, 12.7235) (-0.1838, 12.6697) (-0.2448, 12.622) (-0.3119, 12.5804) (-0.3845, 12.5443) (-0.4467, 12.5194) (-0.4955, 12.5029) (-0.5289, 12.4929) (-0.5459, 12.4881) knots 0 0 0 0 0 0 0.1 0.2 0.3 0.4 0.5 0.6 0.7 0.8 0.9 1 1 1 1 1 1
  spline S46 degree 5 poles (-1.6606, 12.8935) (-1.654, 12.879) (-1.6403, 12.8506) (-1.6187, 12.8094) (-1.5875, 12.7575) (-1.5441, 12.6979) (-1.4961, 12.6441) (-1.443, 12.5966) (-1.3847, 12.5557) (-1.3213, 12.521) (-1.2533, 12.4921) (-1.1954, 12.4733) (-1.1502, 12.4614) (-1.1192, 12.4544) (-1.1036, 12.4512) knots 0 0 0 0 0 0 0.1 0.2 0.3 0.4 0.5 0.6 0.7 0.8 0.9 1 1 1 1 1 1
  spline S47 degree 5 poles (-3.3318, 12.5612) (-3.3338, 12.5446) (-3.3382, 12.5118) (-3.3467, 12.4635) (-3.3614, 12.4012) (-3.3862, 12.3269) (-3.4177, 12.2565) (-3.4567, 12.1904) (-3.5033, 12.1286) (-3.5573, 12.071) (-3.6181, 12.0173) (-3.6717, 11.9772) (-3.7146, 11.9487) (-3.7443, 11.9303) (-3.7594, 11.9213) knots 0 0 0 0 0 0 0.1 0.2 0.3 0.4 0.5 0.6 0.7 0.8 0.9 1 1 1 1 1 1
  point P0 (-7.5478, 10.1896)
  point P1 (-9.0909, 8.8298)
  point P2 (-9.9279, 7.8889)
  point P3 (-11.0665, 6.176)
  point P4 (-11.6314, 5.0505)
  point P5 (-12.2879, 3.1014)
  point P6 (-12.5422, 1.868)
  point P7 (-12.6719, -0.1846)
  point P8 (-12.5983, -1.4418)
  point P9 (-12.1923, -3.4581)
  point P10 (-11.7959, -4.6534)
  point P11 (-10.8818, -6.4958)
  point P12 (-10.1896, -7.5478)
  point P13 (-8.8298, -9.0909)
  point P14 (-7.8889, -9.9279)
  point P15 (-6.176, -11.0665)
  point P16 (-5.0505, -11.6314)
  point P17 (-3.1014, -12.2879)
  point P18 (-1.868, -12.5422)
  point P19 (0.1846, -12.6719)
  point P20 (1.4418, -12.5983)
  point P21 (3.4581, -12.1923)
  point P22 (4.6534, -11.7959)
  point P23 (6.4958, -10.8818)
  point P24 (7.5478, -10.1896)
  point P25 (9.0909, -8.8298)
  point P26 (9.9279, -7.8889)
  point P27 (11.0665, -6.176)
  point P28 (11.6314, -5.0505)
  point P29 (12.2879, -3.1014)
  point P30 (12.5422, -1.868)
  point P31 (12.6719, 0.1846)
  point P32 (12.5983, 1.4418)
  point P33 (12.1923, 3.4581)
  point P34 (11.7959, 4.6534)
  point P35 (10.8818, 6.4958)
  point P36 (10.1896, 7.5478)
  point P37 (8.8298, 9.0909)
  point P38 (7.8889, 9.9279)
  point P39 (6.176, 11.0665)
  point P40 (5.0505, 11.6314)
  point P41 (3.1014, 12.2879)
  point P42 (1.868, 12.5422)
  point P43 (-0.1846, 12.6719)
  point P44 (-1.4418, 12.5983)
  point P45 (-3.4581, 12.1923)
  dimension "d1" = 25
  dimension "d2" = 3
  dimension "d3" = 1.6
  dimension "d4" = 3
  dimension "d5" = 1.7
  dimension "d6" = 1.6
  dimension "d8" = 360
  dimension "d9" = 0.5
  dimension "d10" = 0.5
  dimension "d12" = 360
  dimension "d13" = 0.5
  dimension "d14" = 0.5
  dimension "d15" = 0.1
  dimension "d16" = 0.5
  dimension "d17" = 0.5
  dimension "d18" = 0.1
  dimension "d20" = 360
  constraint coincident A0.centre L0.start
  constraint coincident A0 L0.end
  constraint vertical L0
  constraint parallel L0 L1
  constraint coincident A0 L2.end
  constraint parallel L3 L4
  constraint perpendicular L4 L5
  constraint coincident A0 L6.end
  constraint coincident A0 L7.end
  constraint perpendicular L5 L7
  constraint midpoint L7 L77.end
  constraint midpoint L5 L78.start
  constraint parallel L5 L78
  constraint parallel L5 L79
  constraint midpoint L4 L81.end
  constraint parallel L8 L128
  constraint perpendicular L8 L129
  constraint midpoint L130 L131.start
  constraint perpendicular L130 L131
  constraint coincident A0 S0.end
  constraint parallel L10 L132
  constraint tangent A0 L133
  constraint midpoint L134 L135.start
  constraint perpendicular L134 L135
  constraint coincident A0 S1.end
  measures "d1" diameter of A0
  measures "d2" distance of L0.end L1.end
  measures "d3" distance of L0.end L2.end
  measures "d4" distance of L2.end L4.end
  measures "d5" distance of L4.end L5.end
  measures "d6" distance of L0.end L6.end
  measures "d9" distance of L78.start L78.end
  measures "d10" distance of L78.start L79.end
  measures "d13" distance of L8.start L128.end
  measures "d14" distance of L8.start L129.end
  measures "d15" distance of L131.start L131.end
  measures "d16" distance of L10.end L132.end
  measures "d17" distance of L10.end L133.end
  measures "d18" distance of L135.start L135.end
extrude "Extrude1" add sketch "Sketch1" along normal blind 4 contours A0 L0 L3 L6 | A0 L56 L57 L58 L114 L115 | A0 L58 S33 | A0 L56 S32 | A0 L59 S34 | A0 L55 S31 | A0 L59 L60 L61 L116 L117 | A0 L53 L54 L55 L112 L113 | A0 L61 S35 | A0 L53 S30 | A0 L62 S36 | A0 L52 S29 | A0 L62 L63 L64 L118 L119 | A0 L50 L51 L52 L110 L111 | A0 L64 S37 | A0 L50 S28 | A0 L65 S38 | A0 L49 S27 | A0 L65 L66 L67 L120 L121 | A0 L47 L48 L49 L108 L109 | A0 L67 S39 | A0 L47 S26 | A0 L68 S40 | A0 L46 S25 | A0 L68 L69 L70 L122 L123 | A0 L44 L45 L46 L106 L107 | A0 L70 S41 | A0 L44 S24 | A0 L71 S42 | A0 L43 S23 | A0 L71 L72 L73 L124 L125 | A0 L41 L42 L43 L104 L105 | A0 L73 S43 | A0 L41 S22 | A0 L74 S44 | A0 L40 S21 | A0 L1 L74 L75 L76 L126 L127 | A0 L38 L39 L40 L102 L103 | A0 L6 | A0 L38 S20 | A0 L2 | A0 L1 L76 | L0 L2 L3 | A0 L1 L76 S45 | A0 L4 S46 | A0 L4 L5 L7 L77 L78 L79 L80 L81 | A0 L37 S19 | A0 L7 L77 S47 | A0 L35 L36 L37 L100 L101 | A0 L35 S18 | A0 L8 L9 L10 L82 L83 L128 L132 | L8 L128 L129 S0 | A0 L34 S17 | L10 L132 L133 S1 | A0 L32 L33 L34 L98 L99 | A0 L32 S16 | A0 L11 S2 | A0 L11 L12 L13 L84 L85 | A0 L31 S15 | A0 L13 S3 | A0 L29 L30 L31 L96 L97 | A0 L29 S14 | A0 L14 S4 | A0 L14 L15 L16 L86 L87 | A0 L28 S13 | A0 L16 S5 | A0 L26 L27 L28 L94 L95 | A0 L26 S12 | A0 L17 S6 | A0 L17 L18 L19 L88 L89 | A0 L25 S11 | A0 L19 S7 | A0 L23 L24 L25 L92 L93 | A0 L23 S10 | A0 L20 S8 | A0 L20 L21 L22 L90 L91 | A0 L22 S9
sketch "Sketch2" plane through (0, 4, 0) normal (0, 1, 0) x (-1, 0, 0)
  line L0 (2.3271, -15.3283) -> (3.3189, -15.2006)
  line L1 (3.3189, -15.2006) -> (3.467, -13.6106)
  line L2 (3.467, -13.6106) -> (3.3318, -12.5612)
  spline S0 degree 5 poles (3.3318, -12.5612) (3.3338, -12.5446) (3.3382, -12.5118) (3.3467, -12.4635) (3.3614, -12.4012) (3.3862, -12.3269) (3.4177, -12.2565) (3.4567, -12.1904) (3.5033, -12.1286) (3.5573, -12.071) (3.6181, -12.0173) (3.6717, -11.9772) (3.7146, -11.9487) (3.7443, -11.9303) (3.7594, -11.9213) knots 0 0 0 0 0 0 0.1 0.2 0.3 0.4 0.5 0.6 0.7 0.8 0.9 1 1 1 1 1 1
  arc A0 (3.7594, -11.9213) -> (4.751, -11.5619) centre (0, 0) ccw
  line L3 (4.751, -11.5619) -> (4.3177, -11.74)
  spline S1 degree 5 poles (4.3177, -11.74) (4.3277, -11.7396) (4.3533, -11.7391) (4.3941, -11.7395) (4.4491, -11.7428) (4.517, -11.7524) (4.5872, -11.7695) (4.6541, -11.7939) (4.7177, -11.8261) (4.778, -11.8656) (4.8353, -11.9119) (4.8789, -11.954) (4.9104, -11.9882) (4.931, -12.0121) (4.9411, -12.0244) knots -0.963292 -0.963292 -0.963292 -0.963292 -0.963292 -0.963292 -0.9 -0.8 -0.7 -0.6 -0.5 -0.4 -0.3 -0.2 -0.1 0 0 0 0 0 0
  line L4 (4.9411, -12.0244) -> (5.3212, -12.9493)
  line L5 (5.3212, -12.9493) -> (6.215, -14.2037)
  line L6 (6.215, -14.2037) -> (7.14, -13.8236)
  line L7 (7.14, -13.8236) -> (6.8715, -12.2495)
  line L8 (6.8715, -12.2495) -> (6.4694, -11.2708)
  spline S2 degree 5 poles (6.4694, -11.2708) (6.467, -11.2543) (6.4628, -11.2214) (6.4584, -11.1727) (6.4566, -11.1087) (6.4612, -11.0305) (6.4735, -10.9543) (6.494, -10.8803) (6.523, -10.8086) (6.5603, -10.739) (6.6013, -10.6771) (6.6378, -10.63) (6.6663, -10.5966) (6.6845, -10.5763) (6.6913, -10.569) knots 0 0 0 0 0 0 0.1 0.2 0.3 0.4 0.5 0.6 0.7 0.8 0.9 0.957627 0.957627 0.957627 0.957627 0.957627 0.957627
  line L9 (6.6913, -10.569) -> (6.2793, -10.8083)
  arc A1 (6.2793, -10.8083) -> (7.1813, -10.2313) centre (0, 0) ccw
  spline S3 degree 5 poles (7.1813, -10.2313) (7.1965, -10.2262) (7.2268, -10.2168) (7.2719, -10.2045) (7.3314, -10.1918) (7.4048, -10.1828) (7.477, -10.1812) (7.548, -10.1875) (7.6177, -10.2021) (7.6862, -10.2246) (7.7535, -10.2546) (7.8066, -10.2839) (7.8459, -10.3088) (7.8719, -10.3266) (7.8849, -10.3358) knots -1 -1 -1 -1 -1 -1 -0.9 -0.8 -0.7 -0.6 -0.5 -0.4 -0.3 -0.2 -0.1 0 0 0 0 0 0
  line L10 (7.8849, -10.3358) -> (8.4914, -11.1309)
  line L11 (8.4914, -11.1309) -> (9.6795, -12.1112)
  line L12 (9.6795, -12.1112) -> (10.4745, -11.5047)
  line L13 (10.4745, -11.5047) -> (9.8078, -10.0536)
  line L14 (9.8078, -10.0536) -> (9.166, -9.2124)
  spline S4 degree 5 poles (9.166, -9.2124) (9.1594, -9.197) (9.1469, -9.1664) (9.1301, -9.1204) (9.1117, -9.0591) (9.096, -8.9823) (9.0881, -8.9056) (9.0888, -8.8288) (9.0982, -8.752) (9.1162, -8.6752) (9.142, -8.5983) (9.1684, -8.5367) (9.1913, -8.4906) (9.2078, -8.4598) (9.2164, -8.4444) knots 0 0 0 0 0 0 0.1 0.2 0.3 0.4 0.5 0.6 0.7 0.8 0.9 1 1 1 1 1 1
  arc A2 (9.2164, -8.4444) -> (9.5847, -8.024) centre (0, 0) ccw
  spline S5 degree 5 poles (9.5847, -8.024) (9.598, -8.0152) (9.6248, -7.9982) (9.6652, -7.9747) (9.7194, -7.9471) (9.788, -7.9194) (9.8573, -7.8991) (9.9276, -7.8868) (9.9987, -7.8828) (10.0706, -7.8869) (10.1434, -7.8984) (10.2022, -7.913) (10.2466, -7.9268) (10.2764, -7.9373) (10.2913, -7.9429) knots -1 -1 -1 -1 -1 -1 -0.9 -0.8 -0.7 -0.6 -0.5 -0.4 -0.3 -0.2 -0.1 0 0 0 0 0 0
  line L15 (10.2913, -7.9429) -> (11.0829, -8.5539)
  line L16 (11.0829, -8.5539) -> (12.4842, -9.1933)
  line L17 (12.4842, -9.1933) -> (13.0952, -8.4016)
  line L18 (13.0952, -8.4016) -> (12.0756, -7.1726)
  line L19 (12.0756, -7.1726) -> (11.238, -6.5261)
  spline S6 degree 5 poles (11.238, -6.5261) (11.2277, -6.513) (11.2076, -6.4867) (11.1795, -6.4466) (11.1459, -6.3921) (11.1109, -6.3221) (11.0834, -6.25) (11.0641, -6.1756) (11.0534, -6.099) (11.0509, -6.0201) (11.0559, -5.9392) (11.0655, -5.8729) (11.0756, -5.8224) (11.0836, -5.7884) (11.0879, -5.7713) knots 0 0 0 0 0 0 0.1 0.2 0.3 0.4 0.5 0.6 0.7 0.8 0.9 1 1 1 1 1 1
  arc A3 (11.0879, -5.7713) -> (11.3348, -5.2699) centre (0, 0) ccw
  spline S7 degree 5 poles (11.3348, -5.2699) (11.3455, -5.2579) (11.3669, -5.2346) (11.3998, -5.2014) (11.4451, -5.1607) (11.5042, -5.1162) (11.5659, -5.0786) (11.6305, -5.0486) (11.6982, -5.0264) (11.7688, -5.0117) (11.842, -5.0039) (11.9026, -5.0029) (11.9491, -5.0047) (11.9806, -5.0071) (11.9964, -5.0086) knots -1 -1 -1 -1 -1 -1 -0.9 -0.8 -0.7 -0.6 -0.5 -0.4 -0.3 -0.2 -0.1 0 0 0 0 0 0
  line L20 (11.9964, -5.0086) -> (12.9192, -5.3939)
  line L21 (12.9192, -5.3939) -> (14.4382, -5.6489)
  line L22 (14.4382, -5.6489) -> (14.8235, -4.7261)
  line L23 (14.8235, -4.7261) -> (13.5206, -3.8028)
  line L24 (13.5206, -3.8028) -> (12.5442, -3.3951)
  spline S8 degree 5 poles (12.5442, -3.3951) (12.5308, -3.3852) (12.5046, -3.3649) (12.4671, -3.3335) (12.4205, -3.2895) (12.3685, -3.2309) (12.3233, -3.1684) (12.2855, -3.1016) (12.2553, -3.0303) (12.2325, -2.9548) (12.2164, -2.8753) (12.2085, -2.8088) (12.2051, -2.7574) (12.2041, -2.7225) (12.2038, -2.7049) knots 0 0 0 0 0 0 0.1 0.2 0.3 0.4 0.5 0.6 0.7 0.8 0.9 1 1 1 1 1 1
  arc A4 (12.2038, -2.7049) -> (12.3126, -2.1566) centre (0, 0) ccw
  spline S9 degree 5 poles (12.3126, -2.1566) (12.3197, -2.1423) (12.3344, -2.1143) (12.3576, -2.0737) (12.3908, -2.0226) (12.4363, -1.9644) (12.4862, -1.9121) (12.5409, -1.8664) (12.6005, -1.8274) (12.6649, -1.7949) (12.7337, -1.7685) (12.7919, -1.7518) (12.8373, -1.7415) (12.8683, -1.7357) (12.884, -1.7331) knots -1 -1 -1 -1 -1 -1 -0.9 -0.8 -0.7 -0.6 -0.5 -0.4 -0.3 -0.2 -0.1 0 0 0 0 0 0
  line L25 (12.884, -1.7331) -> (13.875, -1.8664)
  line L26 (13.875, -1.8664) -> (15.4083, -1.7195)
  line L27 (15.4083, -1.7195) -> (15.5416, -0.7284)
  line L28 (15.5416, -0.7284) -> (14.0441, -0.1738)
  line L29 (14.0441, -0.1738) -> (12.9955, -0.0328)
  spline S10 degree 5 poles (12.9955, -0.0328) (12.98, -0.0266) (12.9494, -0.0138) (12.905, 0.0068) (12.8487, 0.0372) (12.7833, 0.0804) (12.7235, 0.1291) (12.6697, 0.1838) (12.622, 0.2448) (12.5804, 0.3119) (12.5443, 0.3845) (12.5194, 0.4467) (12.5029, 0.4955) (12.4929, 0.5289) (12.4881, 0.5459) knots 0 0 0 0 0 0 0.1 0.2 0.3 0.4 0.5 0.6 0.7 0.8 0.9 1 1 1 1 1 1
  arc A5 (12.4881, 0.5459) -> (12.4512, 1.1036) centre (0, 0) ccw
  spline S11 degree 5 poles (12.4512, 1.1036) (12.4544, 1.1192) (12.4614, 1.1502) (12.4733, 1.1954) (12.4921, 1.2533) (12.521, 1.3213) (12.5557, 1.3847) (12.5966, 1.443) (12.6441, 1.4961) (12.6979, 1.5441) (12.7575, 1.5875) (12.8094, 1.6187) (12.8506, 1.6403) (12.879, 1.654) (12.8935, 1.6606) knots -1 -1 -1 -1 -1 -1 -0.9 -0.8 -0.7 -0.6 -0.5 -0.4 -0.3 -0.2 -0.1 0 0 0 0 0 0
  line L30 (12.8935, 1.6606) -> (13.8853, 1.7883)
  line L31 (13.8853, 1.7883) -> (15.3283, 2.3271)
  line L32 (15.3283, 2.3271) -> (15.2006, 3.3189)
  line L33 (15.2006, 3.3189) -> (13.6106, 3.467)
  line L34 (13.6106, 3.467) -> (12.5612, 3.3318)
  spline S12 degree 5 poles (12.5612, 3.3318) (12.5446, 3.3338) (12.5118, 3.3382) (12.4635, 3.3467) (12.4012, 3.3614) (12.3269, 3.3862) (12.2565, 3.4177) (12.1904, 3.4567) (12.1286, 3.5033) (12.071, 3.5573) (12.0173, 3.6181) (11.9772, 3.6717) (11.9487, 3.7146) (11.9303, 3.7443) (11.9213, 3.7594) knots 0 0 0 0 0 0 0.1 0.2 0.3 0.4 0.5 0.6 0.7 0.8 0.9 1 1 1 1 1 1
  arc A6 (11.9213, 3.7594) -> (11.7413, 4.2886) centre (0, 0) ccw
  spline S13 degree 5 poles (11.7413, 4.2886) (11.7404, 4.3045) (11.7391, 4.3362) (11.7389, 4.383) (11.7421, 4.4438) (11.7524, 4.517) (11.7695, 4.5872) (11.7939, 4.6541) (11.8261, 4.7177) (11.8656, 4.778) (11.9119, 4.8353) (11.954, 4.8789) (11.9882, 4.9104) (12.0121, 4.931) (12.0244, 4.9411) knots -1 -1 -1 -1 -1 -1 -0.9 -0.8 -0.7 -0.6 -0.5 -0.4 -0.3 -0.2 -0.1 0 0 0 0 0 0
  line L35 (12.0244, 4.9411) -> (12.9493, 5.3212)
  line L36 (12.9493, 5.3212) -> (14.2037, 6.215)
  line L37 (14.2037, 6.215) -> (13.8236, 7.14)
  line L38 (13.8236, 7.14) -> (12.2495, 6.8715)
  line L39 (12.2495, 6.8715) -> (11.2708, 6.4694)
  spline S14 degree 5 poles (11.2708, 6.4694) (11.2543, 6.467) (11.2214, 6.4628) (11.1727, 6.4584) (11.1087, 6.4566) (11.0305, 6.4612) (10.9543, 6.4735) (10.8803, 6.494) (10.8086, 6.523) (10.739, 6.5603) (10.6714, 6.6051) (10.6188, 6.6465) (10.5801, 6.6805) (10.5547, 6.7045) (10.542, 6.7168) knots 0 0 0 0 0 0 0.1 0.2 0.3 0.4 0.5 0.6 0.7 0.8 0.9 1 1 1 1 1 1
  arc A7 (10.542, 6.7168) -> (10.2313, 7.1813) centre (0, 0) ccw
  spline S15 degree 5 poles (10.2313, 7.1813) (10.2262, 7.1965) (10.2168, 7.2268) (10.2045, 7.2719) (10.1918, 7.3314) (10.1828, 7.4048) (10.1812, 7.477) (10.1875, 7.548) (10.2021, 7.6177) (10.2246, 7.6862) (10.2546, 7.7535) (10.2839, 7.8066) (10.3088, 7.8459) (10.3266, 7.8719) (10.3358, 7.8849) knots -1 -1 -1 -1 -1 -1 -0.9 -0.8 -0.7 -0.6 -0.5 -0.4 -0.3 -0.2 -0.1 0 0 0 0 0 0
  line L40 (10.3358, 7.8849) -> (11.1309, 8.4914)
  line L41 (11.1309, 8.4914) -> (12.1112, 9.6795)
  line L42 (12.1112, 9.6795) -> (11.5047, 10.4745)
  line L43 (11.5047, 10.4745) -> (10.0536, 9.8078)
  line L44 (10.0536, 9.8078) -> (9.2124, 9.166)
  spline S16 degree 5 poles (9.2124, 9.166) (9.197, 9.1594) (9.1664, 9.1469) (9.1204, 9.1301) (9.0591, 9.1117) (8.9823, 9.096) (8.9056, 9.0881) (8.8288, 9.0888) (8.752, 9.0982) (8.6752, 9.1162) (8.5983, 9.142) (8.5367, 9.1684) (8.4906, 9.1913) (8.4598, 9.2078) (8.4444, 9.2164) knots 0 0 0 0 0 0 0.1 0.2 0.3 0.4 0.5 0.6 0.7 0.8 0.9 1 1 1 1 1 1
  arc A8 (8.4444, 9.2164) -> (8.024, 9.5847) centre (0, 0) ccw
  spline S17 degree 5 poles (8.024, 9.5847) (8.0152, 9.598) (7.9982, 9.6248) (7.9747, 9.6652) (7.9471, 9.7194) (7.9194, 9.788) (7.8991, 9.8573) (7.8868, 9.9276) (7.8828, 9.9987) (7.8869, 10.0706) (7.8984, 10.1434) (7.913, 10.2022) (7.9268, 10.2466) (7.9373, 10.2764) (7.9429, 10.2913) knots -1 -1 -1 -1 -1 -1 -0.9 -0.8 -0.7 -0.6 -0.5 -0.4 -0.3 -0.2 -0.1 0 0 0 0 0 0
  line L45 (7.9429, 10.2913) -> (8.5539, 11.0829)
  line L46 (8.5539, 11.0829) -> (9.1933, 12.4842)
  line L47 (9.1933, 12.4842) -> (8.4016, 13.0952)
  line L48 (8.4016, 13.0952) -> (7.1726, 12.0756)
  line L49 (7.1726, 12.0756) -> (6.5261, 11.238)
  spline S18 degree 5 poles (6.5261, 11.238) (6.513, 11.2277) (6.4867, 11.2076) (6.4466, 11.1795) (6.3921, 11.1459) (6.3221, 11.1109) (6.25, 11.0834) (6.1756, 11.0641) (6.099, 11.0534) (6.0201, 11.0509) (5.9392, 11.0559) (5.8729, 11.0655) (5.8224, 11.0756) (5.7884, 11.0836) (5.7713, 11.0879) knots 0 0 0 0 0 0 0.1 0.2 0.3 0.4 0.5 0.6 0.7 0.8 0.9 1 1 1 1 1 1
  arc A9 (5.7713, 11.0879) -> (5.2699, 11.3348) centre (0, 0) ccw
  spline S19 degree 5 poles (5.2699, 11.3348) (5.2579, 11.3455) (5.2346, 11.3669) (5.2014, 11.3998) (5.1607, 11.4451) (5.1162, 11.5042) (5.0786, 11.5659) (5.0486, 11.6305) (5.0264, 11.6982) (5.0117, 11.7688) (5.0039, 11.842) (5.0029, 11.9026) (5.0047, 11.9491) (5.0071, 11.9806) (5.0086, 11.9964) knots -1 -1 -1 -1 -1 -1 -0.9 -0.8 -0.7 -0.6 -0.5 -0.4 -0.3 -0.2 -0.1 0 0 0 0 0 0
  line L50 (5.0086, 11.9964) -> (5.3939, 12.9192)
  line L51 (5.3939, 12.9192) -> (5.6489, 14.4382)
  line L52 (5.6489, 14.4382) -> (4.7261, 14.8235)
  line L53 (4.7261, 14.8235) -> (3.8028, 13.5206)
  line L54 (3.8028, 13.5206) -> (3.3951, 12.5442)
  spline S20 degree 5 poles (3.3951, 12.5442) (3.3852, 12.5308) (3.3649, 12.5046) (3.3335, 12.4671) (3.2895, 12.4205) (3.2309, 12.3685) (3.1684, 12.3233) (3.1016, 12.2855) (3.0303, 12.2553) (2.9548, 12.2325) (2.8753, 12.2164) (2.8088, 12.2085) (2.7574, 12.2051) (2.7225, 12.2041) (2.7049, 12.2038) knots 0 0 0 0 0 0 0.1 0.2 0.3 0.4 0.5 0.6 0.7 0.8 0.9 1 1 1 1 1 1
  arc A10 (2.7049, 12.2038) -> (2.1566, 12.3126) centre (0, 0) ccw
  spline S21 degree 5 poles (2.1566, 12.3126) (2.1423, 12.3197) (2.1143, 12.3344) (2.0737, 12.3576) (2.0226, 12.3908) (1.9644, 12.4363) (1.9121, 12.4862) (1.8664, 12.5409) (1.8274, 12.6005) (1.7949, 12.6649) (1.7685, 12.7337) (1.7518, 12.7919) (1.7415, 12.8373) (1.7357, 12.8683) (1.7331, 12.884) knots -1 -1 -1 -1 -1 -1 -0.9 -0.8 -0.7 -0.6 -0.5 -0.4 -0.3 -0.2 -0.1 0 0 0 0 0 0
  line L55 (1.7331, 12.884) -> (1.8664, 13.875)
  line L56 (1.8664, 13.875) -> (1.7195, 15.4083)
  line L57 (1.7195, 15.4083) -> (0.7284, 15.5416)
  line L58 (0.7284, 15.5416) -> (0.1738, 14.0441)
  line L59 (0.1738, 14.0441) -> (0.0328, 12.9955)
  spline S22 degree 5 poles (0.0328, 12.9955) (0.0266, 12.98) (0.0138, 12.9494) (-0.0068, 12.905) (-0.0372, 12.8487) (-0.0804, 12.7833) (-0.1291, 12.7235) (-0.1838, 12.6697) (-0.2448, 12.622) (-0.3119, 12.5804) (-0.3845, 12.5443) (-0.4467, 12.5194) (-0.4955, 12.5029) (-0.5289, 12.4929) (-0.5459, 12.4881) knots 0 0 0 0 0 0 0.1 0.2 0.3 0.4 0.5 0.6 0.7 0.8 0.9 1 1 1 1 1 1
  arc A11 (-0.5459, 12.4881) -> (-1.1036, 12.4512) centre (0, 0) ccw
  spline S23 degree 5 poles (-1.1036, 12.4512) (-1.1192, 12.4544) (-1.1502, 12.4614) (-1.1954, 12.4733) (-1.2533, 12.4921) (-1.3213, 12.521) (-1.3847, 12.5557) (-1.443, 12.5966) (-1.4961, 12.6441) (-1.5441, 12.6979) (-1.5875, 12.7575) (-1.6187, 12.8094) (-1.6403, 12.8506) (-1.654, 12.879) (-1.6606, 12.8935) knots -1 -1 -1 -1 -1 -1 -0.9 -0.8 -0.7 -0.6 -0.5 -0.4 -0.3 -0.2 -0.1 0 0 0 0 0 0
  line L60 (-1.6606, 12.8935) -> (-1.7883, 13.8853)
  line L61 (-1.7883, 13.8853) -> (-2.3271, 15.3283)
  line L62 (-2.3271, 15.3283) -> (-3.3189, 15.2006)
  line L63 (-3.3189, 15.2006) -> (-3.467, 13.6106)
  line L64 (-3.467, 13.6106) -> (-3.3318, 12.5612)
  spline S24 degree 5 poles (-3.3318, 12.5612) (-3.3338, 12.5446) (-3.3382, 12.5118) (-3.3467, 12.4635) (-3.3614, 12.4012) (-3.3862, 12.3269) (-3.4177, 12.2565) (-3.4567, 12.1904) (-3.5033, 12.1286) (-3.5573, 12.071) (-3.6181, 12.0173) (-3.6717, 11.9772) (-3.7146, 11.9487) (-3.7443, 11.9303) (-3.7594, 11.9213) knots 0 0 0 0 0 0 0.1 0.2 0.3 0.4 0.5 0.6 0.7 0.8 0.9 1 1 1 1 1 1
  arc A12 (-3.7594, 11.9213) -> (-4.2886, 11.7413) centre (0, 0) ccw
  spline S25 degree 5 poles (-4.2886, 11.7413) (-4.3045, 11.7404) (-4.3362, 11.7391) (-4.383, 11.7389) (-4.4438, 11.7421) (-4.517, 11.7524) (-4.5872, 11.7695) (-4.6541, 11.7939) (-4.7177, 11.8261) (-4.778, 11.8656) (-4.8353, 11.9119) (-4.8789, 11.954) (-4.9104, 11.9882) (-4.931, 12.0121) (-4.9411, 12.0244) knots -1 -1 -1 -1 -1 -1 -0.9 -0.8 -0.7 -0.6 -0.5 -0.4 -0.3 -0.2 -0.1 0 0 0 0 0 0
  line L65 (-4.9411, 12.0244) -> (-5.3212, 12.9493)
  line L66 (-5.3212, 12.9493) -> (-6.215, 14.2037)
  line L67 (-6.215, 14.2037) -> (-7.14, 13.8236)
  line L68 (-7.14, 13.8236) -> (-6.8715, 12.2495)
  line L69 (-6.8715, 12.2495) -> (-6.4694, 11.2708)
  spline S26 degree 5 poles (-6.4694, 11.2708) (-6.467, 11.2543) (-6.4628, 11.2214) (-6.4584, 11.1727) (-6.4566, 11.1087) (-6.4612, 11.0305) (-6.4735, 10.9543) (-6.494, 10.8803) (-6.523, 10.8086) (-6.5603, 10.739) (-6.6051, 10.6714) (-6.6465, 10.6188) (-6.6805, 10.5801) (-6.7045, 10.5547) (-6.7168, 10.542) knots 0 0 0 0 0 0 0.1 0.2 0.3 0.4 0.5 0.6 0.7 0.8 0.9 1 1 1 1 1 1
  arc A13 (-6.7168, 10.542) -> (-7.1813, 10.2313) centre (0, 0) ccw
  spline S27 degree 5 poles (-7.1813, 10.2313) (-7.1965, 10.2262) (-7.2268, 10.2168) (-7.2719, 10.2045) (-7.3314, 10.1918) (-7.4048, 10.1828) (-7.477, 10.1812) (-7.548, 10.1875) (-7.6177, 10.2021) (-7.6862, 10.2246) (-7.7535, 10.2546) (-7.8066, 10.2839) (-7.8459, 10.3088) (-7.8719, 10.3266) (-7.8849, 10.3358) knots -1 -1 -1 -1 -1 -1 -0.9 -0.8 -0.7 -0.6 -0.5 -0.4 -0.3 -0.2 -0.1 0 0 0 0 0 0
  line L70 (-7.8849, 10.3358) -> (-8.4914, 11.1309)
  line L71 (-8.4914, 11.1309) -> (-9.6795, 12.1112)
  line L72 (-9.6795, 12.1112) -> (-10.4745, 11.5047)
  line L73 (-10.4745, 11.5047) -> (-9.8078, 10.0536)
  line L74 (-9.8078, 10.0536) -> (-9.166, 9.2124)
  spline S28 degree 5 poles (-9.166, 9.2124) (-9.1594, 9.197) (-9.1469, 9.1664) (-9.1301, 9.1204) (-9.1117, 9.0591) (-9.096, 8.9823) (-9.0881, 8.9056) (-9.0888, 8.8288) (-9.0982, 8.752) (-9.1162, 8.6752) (-9.142, 8.5983) (-9.1684, 8.5367) (-9.1913, 8.4906) (-9.2078, 8.4598) (-9.2164, 8.4444) knots 0 0 0 0 0 0 0.1 0.2 0.3 0.4 0.5 0.6 0.7 0.8 0.9 1 1 1 1 1 1
  arc A14 (-9.2164, 8.4444) -> (-9.5847, 8.024) centre (0, 0) ccw
  spline S29 degree 5 poles (-9.5847, 8.024) (-9.598, 8.0152) (-9.6248, 7.9982) (-9.6652, 7.9747) (-9.7194, 7.9471) (-9.788, 7.9194) (-9.8573, 7.8991) (-9.9276, 7.8868) (-9.9987, 7.8828) (-10.0706, 7.8869) (-10.1434, 7.8984) (-10.2022, 7.913) (-10.2466, 7.9268) (-10.2764, 7.9373) (-10.2913, 7.9429) knots -1 -1 -1 -1 -1 -1 -0.9 -0.8 -0.7 -0.6 -0.5 -0.4 -0.3 -0.2 -0.1 0 0 0 0 0 0
  line L75 (-10.2913, 7.9429) -> (-11.0829, 8.5539)
  line L76 (-11.0829, 8.5539) -> (-12.4842, 9.1933)
  line L77 (-12.4842, 9.1933) -> (-13.0952, 8.4016)
  line L78 (-13.0952, 8.4016) -> (-12.0756, 7.1726)
  line L79 (-12.0756, 7.1726) -> (-11.238, 6.5261)
  spline S30 degree 5 poles (-11.238, 6.5261) (-11.2277, 6.513) (-11.2076, 6.4867) (-11.1795, 6.4466) (-11.1459, 6.3921) (-11.1109, 6.3221) (-11.0834, 6.25) (-11.0641, 6.1756) (-11.0534, 6.099) (-11.0509, 6.0201) (-11.0559, 5.9392) (-11.0655, 5.8729) (-11.0756, 5.8224) (-11.0836, 5.7884) (-11.0879, 5.7713) knots 0 0 0 0 0 0 0.1 0.2 0.3 0.4 0.5 0.6 0.7 0.8 0.9 1 1 1 1 1 1
  arc A15 (-11.0879, 5.7713) -> (-11.3348, 5.2699) centre (0, 0) ccw
  spline S31 degree 5 poles (-11.3348, 5.2699) (-11.3455, 5.2579) (-11.3669, 5.2346) (-11.3998, 5.2014) (-11.4451, 5.1607) (-11.5042, 5.1162) (-11.5659, 5.0786) (-11.6305, 5.0486) (-11.6982, 5.0264) (-11.7688, 5.0117) (-11.842, 5.0039) (-11.9026, 5.0029) (-11.9491, 5.0047) (-11.9806, 5.0071) (-11.9964, 5.0086) knots -1 -1 -1 -1 -1 -1 -0.9 -0.8 -0.7 -0.6 -0.5 -0.4 -0.3 -0.2 -0.1 0 0 0 0 0 0
  line L80 (-11.9964, 5.0086) -> (-12.9192, 5.3939)
  line L81 (-12.9192, 5.3939) -> (-14.4382, 5.6489)
  line L82 (-14.4382, 5.6489) -> (-14.8235, 4.7261)
  line L83 (-14.8235, 4.7261) -> (-13.5206, 3.8028)
  line L84 (-13.5206, 3.8028) -> (-12.5442, 3.3951)
  spline S32 degree 5 poles (-12.5442, 3.3951) (-12.5308, 3.3852) (-12.5046, 3.3649) (-12.4671, 3.3335) (-12.4205, 3.2895) (-12.3685, 3.2309) (-12.3233, 3.1684) (-12.2855, 3.1016) (-12.2553, 3.0303) (-12.2325, 2.9548) (-12.2164, 2.8753) (-12.2085, 2.8088) (-12.2051, 2.7574) (-12.2041, 2.7225) (-12.2038, 2.7049) knots 0 0 0 0 0 0 0.1 0.2 0.3 0.4 0.5 0.6 0.7 0.8 0.9 1 1 1 1 1 1
  arc A16 (-12.2038, 2.7049) -> (-12.3126, 2.1566) centre (0, 0) ccw
  spline S33 degree 5 poles (-12.3126, 2.1566) (-12.3197, 2.1423) (-12.3344, 2.1143) (-12.3576, 2.0737) (-12.3908, 2.0226) (-12.4363, 1.9644) (-12.4862, 1.9121) (-12.5409, 1.8664) (-12.6005, 1.8274) (-12.6649, 1.7949) (-12.7337, 1.7685) (-12.7919, 1.7518) (-12.8373, 1.7415) (-12.8683, 1.7357) (-12.884, 1.7331) knots -1 -1 -1 -1 -1 -1 -0.9 -0.8 -0.7 -0.6 -0.5 -0.4 -0.3 -0.2 -0.1 0 0 0 0 0 0
  line L85 (-12.884, 1.7331) -> (-13.875, 1.8664)
  line L86 (-13.875, 1.8664) -> (-15.4083, 1.7195)
  line L87 (-15.4083, 1.7195) -> (-15.5416, 0.7284)
  line L88 (-15.5416, 0.7284) -> (-14.0441, 0.1738)
  line L89 (-14.0441, 0.1738) -> (-12.9955, 0.0328)
  spline S34 degree 5 poles (-12.9955, 0.0328) (-12.98, 0.0266) (-12.9494, 0.0138) (-12.905, -0.0068) (-12.8487, -0.0372) (-12.7833, -0.0804) (-12.7235, -0.1291) (-12.6697, -0.1838) (-12.622, -0.2448) (-12.5804, -0.3119) (-12.5443, -0.3845) (-12.5194, -0.4467) (-12.5029, -0.4955) (-12.4929, -0.5289) (-12.4881, -0.5459) knots 0 0 0 0 0 0 0.1 0.2 0.3 0.4 0.5 0.6 0.7 0.8 0.9 1 1 1 1 1 1
  arc A17 (-12.4881, -0.5459) -> (-12.4512, -1.1036) centre (0, 0) ccw
  spline S35 degree 5 poles (-12.4512, -1.1036) (-12.4544, -1.1192) (-12.4614, -1.1502) (-12.4733, -1.1954) (-12.4921, -1.2533) (-12.521, -1.3213) (-12.5557, -1.3847) (-12.5966, -1.443) (-12.6441, -1.4961) (-12.6979, -1.5441) (-12.7575, -1.5875) (-12.8094, -1.6187) (-12.8506, -1.6403) (-12.879, -1.654) (-12.8935, -1.6606) knots -1 -1 -1 -1 -1 -1 -0.9 -0.8 -0.7 -0.6 -0.5 -0.4 -0.3 -0.2 -0.1 0 0 0 0 0 0
  line L90 (-12.8935, -1.6606) -> (-13.8853, -1.7883)
  line L91 (-13.8853, -1.7883) -> (-15.3283, -2.3271)
  line L92 (-15.3283, -2.3271) -> (-15.2006, -3.3189)
  line L93 (-15.2006, -3.3189) -> (-13.6106, -3.467)
  line L94 (-13.6106, -3.467) -> (-12.5612, -3.3318)
  spline S36 degree 5 poles (-12.5612, -3.3318) (-12.5446, -3.3338) (-12.5118, -3.3382) (-12.4635, -3.3467) (-12.4012, -3.3614) (-12.3269, -3.3862) (-12.2565, -3.4177) (-12.1904, -3.4567) (-12.1286, -3.5033) (-12.071, -3.5573) (-12.0173, -3.6181) (-11.9772, -3.6717) (-11.9487, -3.7146) (-11.9303, -3.7443) (-11.9213, -3.7594) knots 0 0 0 0 0 0 0.1 0.2 0.3 0.4 0.5 0.6 0.7 0.8 0.9 1 1 1 1 1 1